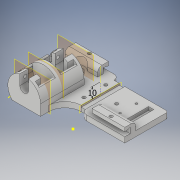
# Autodesk Inventor part: sem2_plate
Saved by Autodesk Inventor 2018 (Build 220112000, 112)
## iProperties
Created: 2018-01-18
Part Number: sem2_plate
Material: Generic
Document SubType Name: Modeling
Designer: rheal
Density: 1 g/cm^3
Appearance: Default
Author: rheal
Autodesk Inventor part; units mm, degrees
ref_plane "YZ Plane" through (0, 0, 0) normal (1, 0, 0) x (0, 1, 0)
ref_plane "XZ Plane" through (0, 0, 0) normal (0, 1, 0) x (-1, 0, 0)
ref_plane "XY Plane" through (0, 0, 0) normal (0, 0, 1) x (1, 0, 0)
sketch "Sketch1" plane through (0, 0, 0) normal (0, 1, 0) x (-1, 0, 0)
  line L0 (60, 37.5) -> (30, 37.5)
  line L1 (60, -17.5) -> (60, 37.5)
  line L2 (60, 37.5) -> (30, 37.5)
  line L3 (-30, 17.5) -> (30, 17.5)
  line L4 (30, 17.5) -> (30, -17.5)
  line L5 (30, -17.5) -> (-30, -17.5)
  line L6 (-30, -17.5) -> (-30, 17.5)
  line L7 (-30, 17.5) -> (30, -17.5) construction
  line L8 (30, 17.5) -> (-30, -17.5) construction
  line L9 (30, 37.5) -> (30, -17.5)
  line L10 (60, -17.5) -> (30, -17.5)
  line L11 (-30, 17.5) -> (30, -17.5)
  point P0 (0, 0)
  dimension "d6" = 30
  constraints: 24 end point, 3 perpendicular, 2 midpoint, 2 parallel, 1 horizontal
  measures "d6" distance of L2.end L0.start
extrude "Extrusion1" add sketch "Sketch1" against normal blind 5
sketch "Sketch2" plane through (-60, 0, 37.5) normal (0, 0, 1) x (1, 0, 0)
  line L0 (30, 0) -> (0, 0) projected
  line L1 (0, 0) -> (0, 5)
  line L2 (0, 5) -> (30, 5)
  line L3 (30, 5) -> (30, 0)
  arc A0 (30, 5) -> (0, 5) centre (15, 5) ccw
  point P0 (60, 0)
  dimension "d10" = 5
  constraints: 6 end point, 2 perpendicular, 2 point on circle, 1 centre point, 1 tangent, 1 vertical
  measures "d10" distance of L0.end L1.end
extrude "Extrusion2" add sketch "Sketch2" against normal blind 35
ref_plane "Work Plane1" through (-60, -5, 32.5) normal (0, 0, 1) x (1, 0, 0)
sketch "Sketch3" plane through (-60, -5, 32.5) normal (0, 0, 1) x (1, 0, 0)
  arc A0 (30, 10) -> (0, 10) centre (15, 10) ccw
  line L0 (15, 25) -> (15, 15)
  line L1 (15, 15) -> (24.5, 15)
  arc A1 (5.5, 15) -> (24.5, 15) centre (15, 15.015626) ccw
  line L2 (5.5, 15) -> (5.5, 21.608187)
  line L3 (24.5, 15) -> (24.5, 21.608187)
  arc A2 (24.5, 21.608187) -> (5.5, 21.608187) centre (15, 10) ccw
  point P0 (60, 5)
  dimension "d14" = 10
  dimension "d16" = 9.5
  dimension "d17" = 19
  constraints: 8 end point, 8 point on circle, 2 centre point, 2 vertical, 1 horizontal, 1 parallel, 1 point on line
  measures "d14" distance of L0.start L0.end
  measures "d16" distance of L0.end L1.end
  measures "d17" distance of L1.end L2.start
extrude "Extrusion3" cut sketch "Sketch3" against normal blind 10
sketch "Sketch4" plane through (-60, -5, 37.5) normal (0, 0, 1) x (1, 0, 0)
  arc A0 (5.5, 15) -> (24.5, 15) centre (15, 15.015626) ccw
  circle A1 centre (15, 15.015626) radius 4
  line L0 (11, 15.015626) -> (11, 24.456832)
  arc A2 (30, 10) -> (0, 10) centre (15, 10) ccw
  line L1 (19, 15.015626) -> (19, 24.456832)
  line L2 (11, 24.456832) -> (8, 24.456832)
  line L3 (8, 24.456832) -> (8, 17.015626)
  line L4 (6, 15.015626) -> (0.863399, 15.015626)
  arc A3 (6, 15.015626) -> (8, 17.015626) centre (6, 17.015626) ccw
  arc A4 (8, 23.266499) -> (0.863399, 15.015626) centre (15, 10) ccw
  line L5 (24.5, 15) -> (22.500195, 15.027962)
  line L6 (22.500195, 15.027962) -> (22.610627, 22.92588)
  line L7 (24.5, 15) -> (24.5, 22.570792)
  line L8 (24.5, 22.570792) -> (22.610627, 22.92588)
  point P0 (60, 5)
  dimension "d20" = 8
  dimension "d21" = 3
  dimension "d22" = 2
  dimension "d60" = 2
  constraints: 18 end point, 11 point on circle, 3 centre point, 3 perpendicular, 3 tangent, 2 vertical, 1 coincident, 1 concentric, 1 horizontal, 1 parallel, 1 point on line
  measures "d20" diameter of A1
  measures "d21" distance of L0.end L2.end
  measures "d22" radius of A3
  measures "d60" distance of L5.start L5.end
extrude "Extrusion4" cut sketch "Sketch4" against normal blind 5 contours A1 | L3 A3 L4 A2 | A1 L0 A2 L1 | L7 L5 L6 A2 | A2 L8 L7
sketch "Sketch5" plane through (-52, 12.015626, 37.5) normal (-1, 0, 0) x (0, 0, 1)
  line L0 (0, -2) -> (0, -6)
  line L1 (0, -6) -> (0, 2)
  line L2 (0, 2) -> (-2.500148, 2)
  line L3 (-5, 7.441207) -> (-5, -2)
  line L4 (-2.500148, 2) -> (-2.500148, 3)
  circle A0 centre (-2.500148, 3) radius 1.5
  point P0 (-37.5, -12.015626)
  dimension "d25" = 8
  dimension "d27" = 1
  dimension "d28" = 3
  constraints: 6 end point, 2 perpendicular, 1 centre point, 1 coincident, 1 collinear
  measures "d25" distance of L0.end L1.end
  measures "d27" distance of L2.end L4.end
  measures "d28" diameter of A0
extrude "Extrusion5" cut sketch "Sketch5" against normal blind 3
ref_plane "Work Plane2" through (-60, -5, 20) normal (0, 0, 1) x (1, 0, 0)
fillet "Fillet1" radius 1 2 edges at (-54.5, 16.6082, 27.5) (-35.5, 16.6082, 30)
mirror "Mirror1" about plane through (-60, -5, 20) normal (0, 0, 1) of "Extrusion4", "Extrusion3", "Fillet1", "Extrusion5"
ref_plane "Work Plane3" through (-60, -5, -7.5) normal (0, 0, 1) x (1, 0, 0)
sketch "Sketch6" plane through (-60, -5, -17.5) normal (-1, 0, 0) x (0, 0, 1)
  line L0 (0, 5) -> (0, 0) projected
  line L1 (5, 5) -> (5, 8.5)
  line L2 (1, 12.5) -> (-5, 12.5)
  arc A0 (5, 8.5) -> (1, 12.5) centre (1, 8.5) ccw
  line L3 (0, 5) -> (0, 10)
  line L4 (-5, 9) -> (0, 10)
  line L5 (-5, 9) -> (-5, 12.5)
  line L6 (0, 5) -> (0, 0) projected
  line L7 (0, 5) -> (5, 5)
  line L8 (0, 5) -> (20, 5) projected
  point P0 (17.5, 5)
  point P1 (5, 12.5)
  dimension "d34" = 10
  dimension "d35" = 7.5
  dimension "d36" = 4
  dimension "d37" = 0
  dimension "d38" = 5
  dimension "d89" = 3.5
  constraints: 12 end point, 2 point on circle, 2 point on line, 2 tangent, 1 centre point, 1 collinear, 1 vertical
  measures "d34" distance of L2.end point (5, 12.5)
  measures "d35" distance of point (5, 12.5) L1.start
  measures "d36" radius of A0
  measures "d37" distance of L0.start L3.start
  measures "d38" distance of L3.start L3.end
  measures "d89" distance of L4.start L2.end
extrude "Extrusion6" add sketch "Sketch6" against normal blind 30
sketch "Sketch7" plane through (-60, 7.5, -16.5) normal (0, 1, 0) x (1, 0, 0)
  line L0 (0, 1) -> (90, 1)
  line L1 (-0.000423, 6.040874) -> (30.000423, 6.041016)
  line L2 (15, 6.040945) -> (15, 3.540945)
  circle A0 centre (15, 3.540945) radius 1.5
  point P0 (60, -16.5)
  dimension "d41" = 30.421
  dimension "d42" = 2.5
  dimension "d43" = 3
  constraints: 4 end point, 1 centre point, 1 coincident, 1 midpoint, 1 vertical
  measures "d41" distance of L0.start L1.end
  measures "d42" distance of L2.start L2.end
  measures "d43" diameter of A0
extrude "Extrusion7" cut sketch "Sketch7" against normal blind 5
sketch "Sketch8" plane through (0, 0, 0) normal (0, 1, 0) x (1, 0, 0)
  line L0 (-30, -17.5) -> (30, -17.5) construction
  line L1 (-30, 17.5) -> (-30, 22.5) construction
  line L2 (-30, -17.5) -> (-30, 22.5) construction
  line L3 (-30, 0) -> (-20, 0) construction
  line L4 (-20, 0) -> (-20, 10) construction
  line L5 (-20, 10) -> (-20, -10) construction
  line L6 (-20, 0) -> (0, 0) construction
  circle A0 centre (-20, 10) radius 1.5
  circle A1 centre (-20, -10) radius 1.5
  circle A2 centre (0, 0) radius 1.5
  dimension "d46" = 10
  dimension "d47" = 10
  dimension "d48" = 20
  dimension "d49" = 3
  dimension "d50" = 3
  dimension "d51" = 3
  constraints: 10 end point, 3 centre point, 3 coincident, 2 horizontal, 2 point on line, 1 perpendicular, 1 vertical
  measures "d46" distance of L3.start L3.end
  measures "d47" distance of L3.end L4.end
  measures "d48" distance of L4.end L5.end
  measures "d49" diameter of A0
  measures "d50" diameter of A1
  measures "d51" diameter of A2
extrude "Extrusion8" cut sketch "Sketch8" against normal blind 5
ref_plane "Work Plane4" through (-15, 0, 17.5) normal (1, 0, 0) x (0, 0, -1)
sketch "Sketch9" plane through (-15, 0, 17.5) normal (1, 0, 0) x (0, 0, -1)
  line L0 (17.5, 0) -> (17.5, 10) construction
  dimension "d55" = 10
  constraints: 2 end point, 1 vertical
  measures "d55" distance of L0.start L0.end
sketch "Sketch10" plane through (-60, -5, 37.5) normal (0, 0, 1) x (1, 0, 0)
  line L0 (0, 0) -> (90, 0)
  line L1 (30, 5) -> (30, 0)
  line L2 (0, 0) -> (30, 0)
  line L3 (30, 10) -> (30, 5)
  line L4 (30, 0) -> (30, 5)
  line L5 (30, 5) -> (0, 5)
  line L6 (0, 10) -> (0, 0)
  line L7 (0, 0) -> (0, 5)
  arc A0 (0.863399, 15.015626) -> (0, 10) centre (15, 10) ccw
  line L8 (19, 24.456832) -> (19, 15.015626)
  arc A1 (30, 10) -> (0.863399, 15.015626) centre (15, 10) ccw
  line L9 (0, 10) -> (0, 5)
  line L10 (30, 5) -> (30, 10)
  arc A2 (11, 15.015626) -> (19, 15.015626) centre (15, 15.015626) ccw
  line L11 (11, 24.456832) -> (11, 15.015626)
  line L12 (11, 15.015626) -> (19, 15.015626)
  line L13 (19, 15.015626) -> (19, 24.456832)
  arc A3 (11, 15.015626) -> (19, 15.015626) centre (15, 15.015626) ccw
  point P0 (60, 5)
  point P1 (72, 0)
  constraints: 18 end point, 5 point on circle, 4 collinear, 4 tangent, 2 centre point, 2 perpendicular, 1 midpoint, 1 parallel, 1 vertical
extrude "Extrusion10" add sketch "Sketch10" along normal blind 2.5 contours L6 L5 L1 L0 | L6 A0 A1 L11 A2 L8 L3 L5
mirror "Mirror4" about plane through (-60, -5, 20) normal (0, 0, 1) of "Extrusion10"
sketch "Sketch12" plane through (-30, 5, -17.5) normal (0, 0, -1) x (-1, 0, 0)
  line L0 (30, -5) -> (0, -5) projected
  line L1 (0, -10) -> (30, -10)
  line L2 (30, -10) -> (30, -5)
  line L3 (30, -5) -> (0, -5)
  line L4 (0, -10) -> (-10, -10)
  line L5 (30, -10) -> (-60, -10) projected
  line L6 (-10, -10) -> (-10, -5)
  line L7 (-10, -5) -> (0, -5)
  point P0 (-30, -5)
  dimension "d116" = 10
  constraints: 12 end point, 3 perpendicular, 1 horizontal, 1 parallel, 1 point on line
  measures "d116" distance of L1.start L4.end
extrude "Extrusion12" add sketch "Sketch12" along normal blind 5
fillet "Fillet3" radius 2 1 edges at (30, -2.5, -17.5)
fillet "Fillet3" radius 15 1 edges at (-30, -2.5, 17.5)
sketch "Sketch15" plane through (-60, 4, -22.5) normal (-1, 0, 0) x (0, 0, 1)
  line L0 (0, -9) -> (62.5, -9)
  line L1 (0, -9) -> (3.41987, -9) construction
  point P0 (22.5, -4)
  constraints: 2 end point, 1 horizontal
pattern_circular "Circular Pattern3" count 2 over 360 about axis through (-15, 0, 0) along (0, 1, 0) of "Extrusion12", "Extrusion6", "Extrusion7"
sketch "Sketch16" plane through (-60, 7.5, -16.5) normal (0, 1, 0) x (1, 0, 0)
  line L0 (19, -16.5) -> (11, -16.5) projected
  line L1 (15, -16.5) -> (15, -1.5)
  circle A0 centre (15, -9) radius 7.5
  point P0 (60, -16.5)
  dimension "d95" = 15
  constraints: 2 end point, 2 midpoint, 1 vertical, 1 vertical alignment, 2 other
  measures "d95" distance of L1.start L1.end
extrude "Extrusion15" cut sketch "Sketch16" against normal blind 7.5
ref_plane "Work Plane5" through (0, -7, 0) normal (0, -1, 0) x (1, 0, 0)
fillet "Fillet7" radius 5 2 edges at (-10, -2.5, 22.5) (-20, -2.5, -22.5)
sketch "Sketch19" plane through (-60, -5, 40) normal (0, 0, 1) x (1, 0, 0)
  point P0 (60, 5)
sketch "Sketch20" plane through (-60, -5, 40) normal (0, 0, 1) x (1, 0, 0)
  line L0 (0, 10) -> (30, 10)
  line L1 (0, 0) -> (0, -2)
  line L2 (0, 0) -> (3.81966, 0)
  line L3 (0, 0) -> (30, 0)
  line L4 (0, 10) -> (0, 5)
  line L5 (0, 0) -> (0, 10)
  arc A0 (0, 10) -> (3.81966, 0) centre (15, 10) ccw
  circle A1 centre (15, 10) radius 15
  line L6 (3, -3.5) -> (18.5, -3.5)
  line L7 (8.461652, -3.5) -> (0, -3.5)
  line L8 (0, -3.5) -> (0, 0)
  point P0 (60, 5)
  constraints: 9 end point, 4 point on circle, 2 centre point, 2 collinear, 2 point on line, 1 coincident, 1 midpoint, 1 perpendicular, 1 tangent
extrude "Extrusion18" cut sketch "Sketch20" against normal through all contours A0 L2 L5 L4 | A1 L6 L7 L8 L1 L2
sketch "Sketch22" plane through (0, 0, 0) normal (0, 1, 0) x (1, 0, 0)
  line L0 (-59.142136, 12.5) -> (-59.142136, 0)
  line L1 (-59.142136, 0) -> (-30, 0)
  arc A0 (-39.40983, 12.5) -> (-50.59017, 12.5) centre (-45, 7.5) ccw
  line L2 (-59.142136, 0) -> (-45, 7.5)
  line L3 (-45, 7.5) -> (-59.142136, 12.5)
  line L4 (-59.142136, 12.5) -> (-59.142136, 0)
  line L5 (-59.142136, 0) -> (-52.071068, 0)
  line L6 (-52.071068, 0) -> (-52.071068, 12.5)
  line L7 (-52.071068, 12.5) -> (-59.142136, 12.5)
  arc A1 (-52.071068, 0) -> (-52.071068, 12.5) centre (-51.187184, 6.25) ccw
  point P0 (0, 0)
  constraints: 12 end point, 3 perpendicular, 3 point on circle, 1 centre point, 1 collinear
extrude "Extrusion20" cut sketch "Sketch22" against normal through all
sketch "Sketch23" plane through (0, -5, 0) normal (0, -1, 0) x (1, 0, 0)
  point P0 (0, 0)
sketch "Sketch24" plane through (28, -5, -17.5) normal (0, 0, -1) x (-1, 0, 0)
  line L0 (48, 0) -> (48, 5) projected
  line L1 (43, 5) -> (38, 5)
  line L2 (38, 5) -> (38, 3.5)
  line L3 (38, 3.5) -> (43, 3.5)
  line L4 (43, 3.5) -> (43, 5)
  point P0 (28, 5)
  dimension "d125" = 5
  dimension "d126" = 1.5
  constraints: 8 end point, 2 parallel, 1 horizontal, 1 perpendicular
  measures "d125" distance of L3.end L2.end
  measures "d126" distance of L2.end L1.end
extrude "Extrusion21" cut sketch "Sketch24" against normal through all
sketch "Sketch25" plane through (0, 0, 0) normal (0, 1, 0) x (1, 0, 0)
  line L0 (16.85331, 12.5) -> (21.696893, 12.5)
  line L1 (21.696893, 12.5) -> (21.696893, -9)
  line L2 (21.696893, -9) -> (16.85331, -9)
  line L3 (28, 17.5) -> (-10, 17.5)
  circle A0 centre (9, 9.223983) radius 1
  circle A1 centre (9, -5.776017) radius 1
  line L4 (16.85331, 12.5) -> (16.85331, -9)
  point P0 (0, 0)
  dimension "d130" = 21.5
  dimension "d131" = 5
  dimension "d132" = 2
  dimension "d133" = 2
  dimension "d134" = 15
  constraints: 8 end point, 2 centre point, 2 perpendicular, 1 horizontal, 1 parallel
  measures "d130" distance of L0.end L1.end
  measures "d131" distance from line of L3 L0.end
  measures "d132" diameter of A0
  measures "d133" diameter of A1
  measures "d134" distance of A1.centre A0.centre
extrude "Extrusion22" cut sketch "Sketch25" against normal blind 3
sketch "Sketch26" plane through (0, 0, 0) normal (0, 1, 0) x (1, 0, 0)
  line L0 (-50.639053, 12.659764) -> (-43.043195, 12.659764)
  line L1 (-43.043195, 0) -> (-50.639053, 0)
  line L2 (-50.639053, 0) -> (-50.639053, 12.659764)
  line L3 (-49, 0) -> (-60, 0)
  arc A0 (-43.043195, 0) -> (-43.043195, 12.659764) centre (-44.690423, 6.329882) ccw
  point P0 (0, 0)
  point P1 (-56.18034, 0)
  dimension "d139" = 0
  constraints: 6 end point, 2 point on circle, 1 centre point, 1 horizontal, 1 parallel
  measures "d139" distance from line of L3 L1.end
extrude "Extrusion23" cut sketch "Sketch26" against normal blind 6
body "Solid1"
